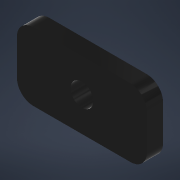
# Autodesk Inventor part: mount_linear_stepper_washer
Saved by Autodesk Inventor 2021 (Build 250183000, 183)
## iProperties
Created: 2020-12-29
Part Number: mount_linear_stepper_washer
Material: ABS Plastic
Document SubType Name: Modeling
Designer: Tomasz
Density: 1.06 g/cm^3
Appearance: Smooth - Black
Author: Tomasz
Autodesk Inventor part; units mm, degrees
ref_plane "YZ Plane" through (0, 0, 0) normal (1, 0, 0) x (0, 1, 0)
ref_plane "XZ Plane" through (0, 0, 0) normal (0, 1, 0) x (-1, 0, 0)
ref_plane "XY Plane" through (0, 0, 0) normal (0, 0, 1) x (1, 0, 0)
sketch "washer_sketch" plane through (0, 0, 0) normal (0, 0, 1) x (1, 0, 0)
  arc A0 (0.0668, 4.8898) -> (-1.1152, 4.3995) centre (0.2018, 2.8944) ccw construction
  line L0 (-7.8667, -1.508) -> (-1.1152, 4.3995) construction
  arc A1 (-7.8667, -1.508) -> (-8.5497, -3.0131) centre (-6.5497, -3.0131) ccw construction
  line L1 (-8.5497, -4.8898) -> (-8.5497, -3.0131) construction
  line L2 (8.5497, -4.8898) -> (-8.5497, -4.8898) construction
  line L3 (1.5081, 4.1255) -> (8.5497, -4.8898) construction
  arc A2 (1.5081, 4.1255) -> (0.0668, 4.8898) centre (-0.0681, 2.8944) ccw construction
  circle A3 centre (-0.4046, -0.6987) radius 3.55 construction
  circle A4 centre (-0.4046, -0.6987) radius 3.55 construction
  circle A5 centre (-0.4046, -0.6987) radius 1.4 projected
  line L4 (-6.4046, -4.8898) -> (5.5954, -4.8898)
  line L5 (7.5954, -2.8898) -> (7.5954, 1.4924)
  line L6 (5.5954, 3.4924) -> (-6.4046, 3.4924)
  line L7 (-8.4046, 1.4924) -> (-8.4046, -2.8898)
  arc A6 (-8.4046, -2.8898) -> (-6.4046, -4.8898) centre (-6.4046, -2.8898) ccw
  arc A7 (-6.4046, 3.4924) -> (-8.4046, 1.4924) centre (-6.4046, 1.4924) ccw
  arc A8 (7.5954, 1.4924) -> (5.5954, 3.4924) centre (5.5954, 1.4924) ccw
  arc A9 (5.5954, -4.8898) -> (7.5954, -2.8898) centre (5.5954, -2.8898) ccw
  point P0 (0, 0)
  point P1 (-8.4046, -4.8898)
  point P2 (7.5954, 3.4924)
  point P3 (-8.4046, 3.4924)
  dimension "d0" = 16
  dimension "d1" = 8
  dimension "d2" = 4.1911
  dimension "d3" = 4.1911
  dimension "d4" = 2
  constraints: 8 end point, 8 point on circle, 8 tangent, 6 point on line, 4 centre point, 3 equal radius, 2 parallel, 1 horizontal, 1 horizontal alignment, 1 perpendicular
  measures "d0" distance of point (7.595, 3.492) point (-8.405, 3.492)
  measures "d1" distance from line of A3.centre L7
  measures "d2" distance from line of L4 A4.centre
  measures "d3" distance from line of L6 A4.centre
  measures "d4" radius of A6
extrude "washer" add sketch "washer_sketch" along normal blind 2
equation "\"d1\" = 0.5 * d0"
equation "\"d3\" = d2"
body "Solid1"
